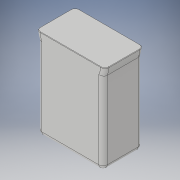
# Autodesk Inventor part: Tc-1
Saved by Autodesk Inventor 2017 (Build 210142000, 142)
## iProperties
Created: 2017-07-13
Part Number: Tc-1
Material: Generic
Document SubType Name: Modeling
Designer: cas7
Density: 1 g/cm^3
Appearance: Default
Author: cas7
Autodesk Inventor part; units mm, degrees
ref_plane "YZ Plane" through (0, 0, 0) normal (1, 0, 0) x (0, 1, 0)
ref_plane "XZ Plane" through (0, 0, 0) normal (0, 1, 0) x (-1, 0, 0)
ref_plane "XY Plane" through (0, 0, 0) normal (0, 0, 1) x (1, 0, 0)
sketch "Sketch1" plane through (0, 0, 0) normal (0, 0, 1) x (1, 0, 0)
  line L0 (0, 0) -> (20, 0)
  line L1 (20, 0) -> (20, 25)
  line L2 (0, 25) -> (0, 0)
  line L3 (0, 27.5) -> (-0.5738, 27.5)
  line L4 (20, 27.5) -> (20.5842, 27.5)
  arc A0 (-0.5738, 27.5) -> (0, 25) centre (7.6984, 28.0827) ccw
  arc A1 (20, 25) -> (20.5842, 27.5) centre (12.3264, 28.1114) ccw
  line L5 (-0.5738, 27.5) -> (20, 27.5)
  dimension "d0" = 20
  dimension "d1" = 25
  constraints: 12 end point, 4 point on circle, 2 centre point, 2 perpendicular, 1 collinear, 1 horizontal, 1 point on line
  measures "d0" distance of L0.start L0.end
  measures "d1" distance of L0.end L1.end
extrude "Extrusion1" add sketch "Sketch1" along normal blind 12
fillet "Fillet1" radius 1.27 12 edges at (10, 0, 12) (20, 12.5, 12) (20, 0, 6) (20, 12.5, 0) (10, 0, 0) (0, 0, 6) (0, 12.5, 0) (0, 12.5, 12) (20.3896, 26.2272, 12) (20.3896, 26.2272, 0) (-0.3841, 26.2277, 0) (-0.3841, 26.2277, 12)
fillet "Fillet2" radius 0.127 7 edges at (-0.2004, 27.5, 11.6285) (-0.5738, 27.5, 6) (-0.2004, 27.5, 0.3715) (19.6696, 27.5, 0.0516) (20.5842, 27.5, 6) (19.6696, 27.5, 11.9484) (10.005, 27.5, 12)
sketch "Sketch2" plane through (1.27, 0, 1.27) normal (0, -1, 0) x (1, 0, 0)
  line L0 (0, 0) -> (-1.27, 0) projected
  line L1 (0, 9.46) -> (0, 10.73) projected
  line L2 (0, 0) -> (0, 9.46)
  circle A0 centre (8.73, 4.73) radius 1.5875
  point P0 (-1.27, -1.27)
  constraints: 2 end point, 1 centre point, 1 collinear
extrude "Extrusion2" cut sketch "Sketch2" against normal blind 1.27
body "Solid1"
